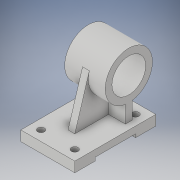
# Autodesk Inventor part: D
Saved by Autodesk Inventor 2018 (Build 220112000, 112)
## iProperties
Created: 2017-09-30
Part Number: D
Material: Generic
Document SubType Name: Modeling
Designer: Soichi
Density: 1 g/cm^3
Appearance: Default
Author: Soichi
Autodesk Inventor part; units mm, degrees
ref_plane "YZ Plane" through (0, 0, 0) normal (1, 0, 0) x (0, 1, 0)
ref_plane "XZ Plane" through (0, 0, 0) normal (0, 1, 0) x (-1, 0, 0)
ref_plane "XY Plane" through (0, 0, 0) normal (0, 0, 1) x (1, 0, 0)
sketch "Sketch1" plane through (0, 0, 0) normal (1, 0, 0) x (0, 1, 0)
  circle A0 centre (0, 0) radius 25
  circle A1 centre (0, 0) radius 35
  line L0 (0, 0) -> (-60, 0) construction
  line L1 (-60, 5) -> (-30, 5)
  line L2 (-30, 5) -> (-30, -5)
  line L3 (-30, -5) -> (-60, -5)
  line L4 (-60, -5) -> (-60, 5)
  line L5 (-60, 90) -> (-75, 90)
  line L6 (-75, 90) -> (-75, -30)
  line L7 (-75, -30) -> (-60, -30)
  line L8 (-60, -30) -> (-60, 90)
  line L9 (-60, -30) -> (-60, 0) construction
  line L10 (-70, 60) -> (-75, 60)
  line L11 (-75, 60) -> (-75, 0)
  line L12 (-75, 0) -> (-70, 0)
  line L13 (-70, 0) -> (-70, 60)
  line L14 (-60, 90) -> (-60, 55) construction
  line L15 (-60, 55) -> (10.2578, 33.4631)
  line L16 (-60, 5) -> (-34.641, 5)
  line L17 (-60, 55) -> (-60, 5)
  point P0 (-75, 30)
  dimension "d0" = 50
  dimension "d1" = 70
  dimension "d2" = 60
  dimension "d3" = 10
  dimension "d4" = 30
  dimension "d5" = 15
  dimension "d6" = 120
  dimension "d7" = 30
  dimension "d8" = 5
  dimension "d9" = 60
  dimension "d10" = 35
  constraints: 36 end point, 6 parallel, 4 horizontal, 3 midpoint, 3 perpendicular, 3 point on line, 2 centre point, 2 coincident, 2 point on circle, 1 collinear, 1 tangent
  measures "d0" diameter of A0
  measures "d1" diameter of A1
  measures "d2" distance of L0.end L0.start
  measures "d3" distance of L1.end L2.end
  measures "d4" distance of L2.end L3.end
  measures "d5" distance of L7.end L6.end
  measures "d6" distance of L6.end L5.end
  measures "d7" distance of L0.end L7.end
  measures "d8" distance of L12.end L11.end
  measures "d9" distance of L11.end L10.end
  measures "d10" distance of L5.start L14.end
extrude "Extrusion1" add sketch "Sketch1" along normal mid plane 60 contours A1 L3 L2 L1 | L3 L4 L1 A1 | A1 L1 L2 L3
extrude "Extrusion2" add sketch "Sketch1" along normal mid plane 10 contours A1 L1 L8 L15
extrude "Extrusion3" add sketch "Sketch1" along normal mid plane 80 contours L8 L4 L7 L6 L12 L13 L10 L5
sketch "Sketch2" plane through (-40, -60, 90) normal (0, 1, 0) x (1, 0, 0)
  line L0 (65, 15) -> (15, 15) construction
  line L1 (40, 15) -> (40, 0) construction
  line L2 (0, 0) -> (80, 0) construction
  line L3 (80, 30) -> (80, 90) construction
  line L4 (80, 60) -> (51.3961, 60) construction
  point P0 (40, 90)
  point P1 (65, 105)
  point P2 (15, 105)
  dimension "d17" = 15
  dimension "d18" = 50
  constraints: 6 end point, 3 midpoint, 2 coincident, 2 horizontal, 2 symmetric about line, 1 vertical
  measures "d17" distance of L1.end L1.start
  measures "d18" distance of L0.start L0.end
hole "Hole1" at (-25, -60, 75) at (-25, -60, -15) at (25, -60, 75) at (25, -60, -15) direction (0, -1, 0) diameter 10 end through all
body "Solid1"
